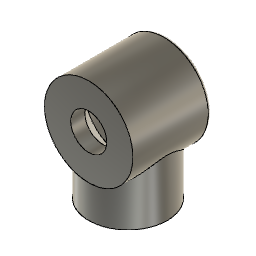
End_Cap_Bolt_CS_Glue v1 (Autodesk Fusion 360 design; units mm, degrees)
Autodesk Fusion 360 part; units mm, degrees
sketch "Sketch1" plane through (0, 0, 0) normal (0, 1, 0) x (1, 0, 0)
  circle A0 centre (0, 0) radius 6.75
  circle A1 centre (0, 0) radius 2.6
  circle A2 centre (0, 0) radius 4.95
  dimension "d1" = 13.5
  dimension "d2" = 5.2
  dimension "d3" = 9.9
  constraint coincident A0.centre A1.centre
  constraint concentric A0 A2
  measures "d1" diameter of A0
  measures "d2" diameter of A1
  measures "d3" diameter of A2
extrude "Extrude1" add sketch "Sketch1" along normal blind 3 contours A0 | A2 makes body 1
extrude "Extrude2" add sketch "Sketch1" along normal blind 12 contours A0 bodies 1
ref_plane "WorkPlane1" through (0, 6.3566, 6.75) normal (0, 0, 1) x (-1, 0, 0)
ref_plane "WorkPlane2" through (0, 2.5583, -6.75) normal (0, 0, -1) x (1, 0, 0)
sketch "Sketch2" plane through (0, 0, 6.75) normal (0, 0, 1) x (1, 0, 0)
  line L0 (6.75, 0) -> (-6.75, 0)
  line L1 (4.95, 3) -> (-4.95, 3)
  circle A0 centre (0.0072, 6) radius 3.937
  line L2 (6.75, 12) -> (-6.75, 12)
  line L3 (-4.95, 12) -> (4.95, 12)
  point P0 (0.0082, 6.3929)
  point P1 (0.0072, 6)
  dimension "d14" = 6
  dimension "d15" = 7.874
  constraint coincident P0
  constraint coincident P1
  constraint coincident P1 A0.centre
  measures "d14" distance of L0 P1
  measures "d15" diameter of A0
sketch "Sketch3" plane through (0, 0, -6.75) normal (0, 0, -1) x (-1, 0, 0)
  line L0 (6.75, 0) -> (-6.75, 0)
  circle A0 centre (0, 6) radius 4.6
  circle A1 centre (0, 6) radius 6
  line L1 (6.75, 11.4938) -> (-6.75, 11.4938)
  point P0 (0, 6)
  dimension "d16" = 6
  dimension "d17" = 9.2
  dimension "d18" = 12
  constraint coincident P0 A0.centre
  constraint concentric A0 A1
  measures "d16" distance of L0 P0
  measures "d17" diameter of A0
  measures "d18" diameter of A1
extrude "Extrude3" add sketch "Sketch3" along normal blind 5 separate body contours A1 L1 picked at (0.1146, 11.1916) makes body 2
extrude "Extrude4" add 1 faces at (-0.1146, 11.1916, -6.75) along direction (0, 0, 1) blind 4 on bodies 2 bodies 2 1
sketch "Sketch4" plane through (0, 12, 0) normal (0, 1, 0) x (-1, 0, 0)
  circle A0 centre (0, 0) radius 4.95
  circle A1 centre (0, 0) radius 6.75
extrude "Extrude5" cut sketch "Sketch4" against normal up to surface (9 mm away) contours A0 bodies 2
extrude "Extrude6" add 3 faces at (2.6875, 3, -2.9182) (-3.708, 3, -3.0137) (3.708, 3, -3.0137) along direction (0, 1, 0) blind 2 on bodies 2 bodies 2
sketch "Sketch5" plane through (0, 5, 0) normal (0, 1, 0) x (-1, 0, 0)
  circle A0 centre (0, 0) radius 2.6
  circle A1 centre (0, 0) radius 4.95
  constraint coincident A0.centre A1.centre
hole "Hole1" at (0, 5, 0) direction (0, -1, 0) diameter 5.5 depth 25.5 tip angle 118 countersink diameter 11.2 countersink angle 90 bodies 2
sketch "Sketch6" plane through (0, 12, 0) normal (0, 1, 0) x (-1, 0, 0)
  circle A0 centre (0, 0) radius 4.95
  circle A1 centre (0, 0) radius 6.75
  circle A2 centre (0, 0) radius 5.6
  dimension "d36" = 11.2
  constraint coincident A0.centre A1.centre
  measures "d36" diameter of A2
extrude "Extrude7" cut sketch "Sketch6" against normal blind 7 contours A2 bodies 2
fillet "Fillet3" radius 0.5 1 edges at (5.221, 12, 2.025) on bodies 2
fillet "Fillet3" radius 0.5 1 edges at (-6.2932, 12, 2.4409) on bodies 2
equation "d15 = ( 25.4 * 0.31 ) * 1 mm"
